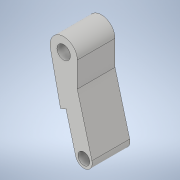
# Autodesk Inventor part: Fangklinke
Saved by Autodesk Inventor 2021 (Build 250183000, 183)
## iProperties
Created: 2021-03-08
Part Number: Fangklinke
Material: Generic
Document SubType Name: Modeling
Designer: Lukas
Density: 1 g/cm^3
Appearance: Default
Author: Lukas
Autodesk Inventor part; units mm, degrees
ref_plane "YZ Plane" through (0, 0, 0) normal (1, 0, 0) x (0, 1, 0)
ref_plane "XZ Plane" through (0, 0, 0) normal (0, 1, 0) x (-1, 0, 0)
ref_plane "XY Plane" through (0, 0, 0) normal (0, 0, 1) x (1, 0, 0)
sketch "Sketch1" plane through (0, 0, 0) normal (0, 0, 1) x (1, 0, 0)
  circle A0 centre (0, 0) radius 3.25
  circle A1 centre (0, 0) radius 1.6
  line L0 (-3.1777, -0.6816) -> (-0.75, -12)
  line L1 (3.25, -6) -> (3.25, 0)
  line L2 (3.25, -6) -> (7.2692, -21)
  line L3 (7.2692, -21) -> (3.4055, -22.0353)
  line L4 (3.4055, -22.0353) -> (0.5726, -11.4628)
  line L5 (0.5726, -11.4628) -> (-0.75, -12)
  circle A2 centre (4.8197, -19.5858) radius 1.4
  dimension "d0" = 6.5
  dimension "d1" = 3.2
  dimension "d3" = 12
  dimension "d24" = 4
  dimension "d26" = 6
  dimension "d31" = 15
  dimension "d32" = 21
  dimension "d33" = 80
  dimension "d34" = 2
  dimension "d35" = 4
  dimension "d36" = 2
  dimension "d37" = 2.8
  constraints: 12 end point, 3 centre point, 2 coincident, 2 point on circle, 2 tangent, 1 parallel, 1 perpendicular, 1 vertical
  measures "d0" diameter of A0
  measures "d1" diameter of A1
  measures "d3" vertical distance of point (0, 0) L0.end
  measures "d24" horizontal distance of L1.start L0.end
  measures "d26" vertical distance of L1.start L0.end
  measures "d31" angle of L2 L1
  measures "d32" vertical distance of L2.end point (0, 0)
  measures "d33" angle of L0 L5
  measures "d34" distance from line of L2 A2.centre
  measures "d35" distance between parallel lines of L4 L2
  measures "d36" distance from line of L3 A2.centre
  measures "d37" diameter of A2
extrude "Extrusion1" add sketch "Sketch1" along normal blind 9
fillet "Fillet5" radius 2 2 edges at (7.2692, -21, 4.5) (3.4055, -22.0353, 4.5)
equation "\"d34\" = 0.5 * d35"
body "Solid1"
